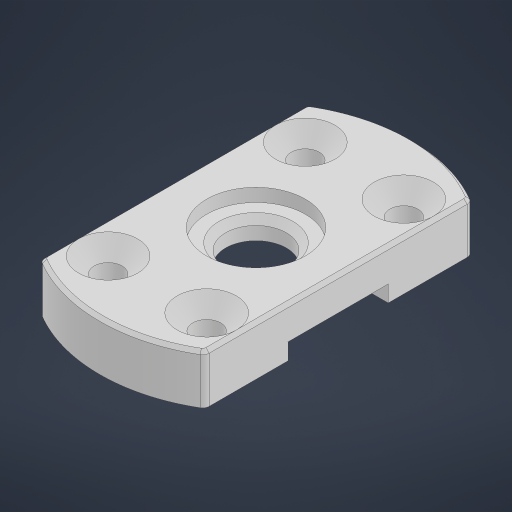
# Autodesk Inventor part: HM1_FIXT2-002
Saved by Autodesk Inventor 2024.3 (Build 283343000, 343)
## iProperties
Created: 2024-10-19
Part Number: HM1_FIXT2-002
Material: Generic
Document SubType Name: Modeling
Designer: fablabadmin
Density: 1 g/cm^3
Appearance: Default
Author: fablabadmin
Autodesk Inventor part; units mm, degrees
ref_plane "YZ Plane" through (0, 0, 0) normal (1, 0, 0) x (0, 1, 0)
ref_plane "XZ Plane" through (0, 0, 0) normal (0, 1, 0) x (-1, 0, 0)
ref_plane "XY Plane" through (0, 0, 0) normal (0, 0, 1) x (1, 0, 0)
sketch "Sketch2" plane through (0, 0, 0) normal (0, 1, 0) x (-1, 0, 0)
  circle A0 centre (0, 0) radius 47.5
  line L0 (25, -40.3887) -> (25, 40.3887)
  line L1 (66.5, 0) -> (-66.5, 0) construction
  line L2 (0, -66.5) -> (0, 66.5) construction
  line L3 (-25, -40.3887) -> (-25, 40.3887)
  dimension "d3" = 95
  dimension "d4" = 50
  constraints: 4 end point, 2 point on circle, 2 symmetric about line, 1 centre point, 1 coincident, 1 vertical
  measures "d3" diameter of A0
  measures "d4" distance between parallel lines of L3 L0
extrude "Extrusion2" add sketch "Sketch2" along normal mid plane 15 contours L0 A0 L3
sketch "Sketch3" plane through (0, -7.5, 0) normal (0, -1, 0) x (1, 0, 0)
  arc A0 (-25, -40.3887) -> (25, -40.3887) centre (0, 0) ccw projected
  line L0 (25, -40.3887) -> (25, 40.3887) projected
  arc A1 (25, 40.3887) -> (-25, 40.3887) centre (0, 0) ccw projected
  line L1 (-25, 40.3887) -> (-25, -40.3887) projected
  line L2 (-25, -15.25) -> (25, -15.25)
  line L3 (25, -15.25) -> (25, 15.25)
  line L4 (25, 15.25) -> (-25, 15.25)
  line L5 (-25, 15.25) -> (-25, -15.25)
  line L6 (-25, -15.25) -> (25, 15.25) construction
  line L7 (25, -15.25) -> (-25, 15.25) construction
  circle A2 centre (0, 0) radius 9.25
  dimension "d7" = 30.5
  dimension "d10" = 18.5
  constraints: 12 end point, 2 midpoint, 2 parallel, 1 centre point, 1 coincident, 1 horizontal, 1 perpendicular, 1 point on line
  measures "d7" distance between parallel lines of L2 L4
  measures "d10" diameter of A2
extrude "Extrusion3" cut sketch "Sketch3" against normal blind 5 contours L1 L4 L0 L2 | A2
extrude "Extrusion4" cut sketch "Sketch3" against normal through all contours A2
sketch "Sketch4" plane through (0, 7.5, 0) normal (0, 1, 0) x (1, 0, 0)
  circle A0 centre (0, 0) radius 15
  dimension "d13" = 30
  constraints: 1 centre point, 1 coincident
  measures "d13" diameter of A0
extrude "Extrusion5" cut sketch "Sketch4" against normal blind 4
chamfer "Chamfer1" distance 2 angle 45 1 edges at (-9.25, 3.5, 0)
sketch "Sketch5" plane through (0, 7.5, 0) normal (0, 1, 0) x (1, 0, 0)
  line L0 (15, -30) -> (-15, -30) construction
  line L1 (-15, -30) -> (-15, 30) construction
  line L2 (-15, 30) -> (15, 30) construction
  line L3 (15, 30) -> (15, -30) construction
  line L4 (15, -30) -> (-15, 30) construction
  line L5 (-15, -30) -> (15, 30) construction
  point P0 (0, 0)
  dimension "d19" = 30
  dimension "d20" = 60
  constraints: 12 end point, 4 coincident, 2 midpoint, 2 parallel, 1 horizontal, 1 perpendicular
  measures "d19" distance of L1.end L2.end
  measures "d20" distance of L0.end L1.end
hole "Hole1" at (-15, 7.5, -30) at (15, 7.5, -30) at (-15, 7.5, 30) at (15, 7.5, 30) direction (0, -1, 0) diameter 8.5 end through all countersink diameter 18 countersink angle 90 clearance for "Countersunk Flat Head Screw ISO 2009/7046" size "M8" standard "ISO"
fillet "Fillet1" radius 2 4 edges at (25, 0, 40.3887) (-25, 0, 40.3887) (-25, 0, -40.3887) (25, 0, -40.3887)
chamfer "Chamfer2" distance 1 angle 45 8 edges at (0, 7.5, 47.5) (24.7352, 7.5, 40.2532) (25, 7.5, 0) (24.7352, 7.5, -40.2532) (0, 7.5, -47.5) (-24.7352, 7.5, -40.2532) (-25, 7.5, 0) (-24.7352, 7.5, 40.2532)
body "Solid2"
